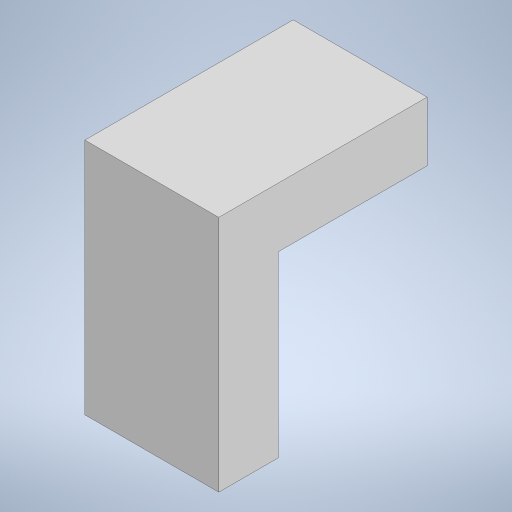
# Autodesk Inventor part: montaz_silniki
Saved by Autodesk Inventor 2023.5 (Build 275446000, 446)
## iProperties
Created: 2025-03-17
Part Number: montaz_silniki
Material: Ogólny
Document SubType Name: Modeling
Designer: kamil
Density: 1 g/cm^3
Appearance: Domyślna
Author: kamil
Autodesk Inventor part; units mm, degrees
ref_plane "YZ Plane" through (0, 0, 0) normal (1, 0, 0) x (0, 1, 0)
ref_plane "XZ Plane" through (0, 0, 0) normal (0, 1, 0) x (-1, 0, 0)
ref_plane "XY Plane" through (0, 0, 0) normal (0, 0, 1) x (1, 0, 0)
sketch "Szkic1" plane through (0, 0, 0) normal (1, 0, 0) x (0, 1, 0)
  line L0 (0, 0) -> (12, 0)
  line L1 (12, 0) -> (12, -10)
  line L2 (16, -10) -> (16, 4)
  line L3 (16, 4) -> (0, 4)
  line L4 (0, 4) -> (0, 0)
  line L5 (12, -10) -> (16, -10)
  dimension "d0" = 12
  dimension "d1" = 10
  dimension "d2" = 4
  constraints: 12 end point, 3 perpendicular, 1 horizontal, 1 vertical, 1 other
  measures "d0" distance of L0.start L0.end
  measures "d1" distance of L0.end L1.end
  measures "d2" distance between parallel lines of L1 L2
extrude "Wyciągnięcie proste1" add sketch "Szkic1" along normal blind 9
